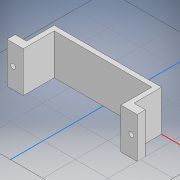
# Autodesk Inventor part: 000.001.013 - Скобе прижима турбины
Saved by Autodesk Inventor 2022 (Build 260153000, 153)
## iProperties
Created: 2023-04-23
Part Number: 000.001.013 - Скобе прижима турбины
Material: Типовые
Document SubType Name: Modeling
Designer: Иван Петров
Density: 1 g/cm^3
Appearance: По умолчанию
Author: Иван Петров
Autodesk Inventor part; units mm, degrees
ref_plane "YZ Plane" through (0, 0, 0) normal (1, 0, 0) x (0, 1, 0)
ref_plane "XZ Plane" through (0, 0, 0) normal (0, 1, 0) x (-1, 0, 0)
ref_plane "XY Plane" through (0, 0, 0) normal (0, 0, 1) x (1, 0, 0)
sketch "Эскиз1" plane through (0, 0, 0) normal (0, 0, 1) x (1, 0, 0)
  line L0 (-30, -12.5) -> (30, -12.5)
  line L1 (30, -12.5) -> (30, 12.5)
  line L2 (30, 12.5) -> (-30, 12.5)
  line L3 (-30, 12.5) -> (-30, -12.5)
  line L4 (-30, -12.5) -> (30, 12.5) construction
  line L5 (30, -12.5) -> (-30, 12.5) construction
  point P0 (0, 0)
  dimension "d0" = 60
  dimension "d14" = 25
  constraints: 12 end point, 2 midpoint, 2 parallel, 1 horizontal, 1 perpendicular
  measures "d0" distance of L2.end L1.end
  measures "d14" distance of L0.end L1.end
extrude "Выдавливание1" add sketch "Эскиз1" along normal blind 3
sketch "Эскиз2" plane through (0, 0, 3) normal (0, 0, 1) x (1, 0, 0)
  line L0 (-30, 12.5) -> (-30, -12.5) projected
  line L1 (-30, 12.5) -> (-33, 12.5)
  line L2 (-33, 12.5) -> (-33, -12.5)
  line L3 (-33, -12.5) -> (-30, -12.5)
  line L4 (-30, -12.5) -> (-30, 12.5)
  point P0 (0, 0)
  dimension "d3" = 3
  constraints: 8 end point, 2 parallel, 1 horizontal, 1 horizontal alignment, 1 perpendicular
  measures "d3" distance of L3.end L2.end
extrude "Выдавливание2" add sketch "Эскиз2" along normal blind 19 and the other way blind 3
sketch "Эскиз3" plane through (0, 0, 22) normal (0, 0, 1) x (1, 0, 0)
  line L0 (-30, -12.5) -> (-30, 12.5) projected
  line L1 (-30, 12.5) -> (-40, 12.5)
  line L2 (-40, 12.5) -> (-40, -12.5)
  line L3 (-40, -12.5) -> (-30, -12.5)
  line L4 (-30, -12.5) -> (-30, 12.5)
  point P0 (0, 0)
  dimension "d8" = 10
  constraints: 8 end point, 2 parallel, 1 horizontal, 1 horizontal alignment, 1 perpendicular
  measures "d8" distance of L3.end L2.end
extrude "Выдавливание3" add sketch "Эскиз3" against normal blind 5
sketch "Эскиз4" plane through (0, 0, 17) normal (0, 0, -1) x (-1, 0, 0)
  circle A0 centre (36.404, 0) radius 1.5
  line L0 (40, -12.5) -> (40, 12.5) projected
  point P0 (0, 0)
  point P1 (40, 0)
  dimension "d11" = 3
  constraints: 1 centre point, 1 horizontal alignment, 1 midpoint
  measures "d11" diameter of A0
extrude "Выдавливание4" cut sketch "Эскиз4" against normal blind 5
mirror "Зеркальное отражение1" about plane through (0, 0, 0) normal (1, 0, 0) of "Выдавливание2", "Выдавливание3", "Выдавливание4"
